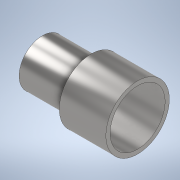
# Autodesk Inventor part: Front Nozzle
Saved by Autodesk Inventor 2021 (Build 250183000, 183)
## iProperties
Created: 2020-04-18
Part Number: Front Nozzle
Material: Generic
Document SubType Name: Modeling
Designer: James
Density: 1 g/cm^3
Appearance: Semi-Polished
Author: James
Autodesk Inventor part; units mm, degrees
ref_plane "YZ Plane" through (0, 0, 0) normal (1, 0, 0) x (0, 1, 0)
ref_plane "XZ Plane" through (0, 0, 0) normal (0, 1, 0) x (-1, 0, 0)
ref_plane "XY Plane" through (0, 0, 0) normal (0, 0, 1) x (1, 0, 0)
sketch "Sketch1" plane through (0, 0, 0) normal (0, 0, 1) x (1, 0, 0)
  line L0 (0, 0) -> (80, 0)
  line L1 (60, 15) -> (60, 11)
  line L2 (60, 11) -> (37, 11)
  line L3 (37, 11) -> (37, 9)
  line L4 (37, 9) -> (62, 9)
  line L5 (62, 9) -> (62, 9)
  line L6 (60, 15) -> (82, 15)
  line L7 (62, 9) -> (62, 13)
  line L8 (62, 13) -> (82, 13)
  line L9 (82, 13) -> (82, 15)
  point P0 (62, 11)
  dimension "d0" = 80
  dimension "d4" = 23
  dimension "d5" = 2
  dimension "d9" = 2
  dimension "d14" = 9
  dimension "d15" = 11
  dimension "d17" = 15
  dimension "d18" = 13
  constraints: 20 end point, 2 horizontal, 2 point on line, 2 vertical
  measures "d0" distance of L0.start L0.end
  measures "d4" distance of L1.end L2.end
  measures "d5" distance of L2.end L3.end
  measures "d9" distance between parallel lines of L5 L1
  measures "d14" distance between parallel lines of L0 L4
  measures "d15" distance between parallel lines of L0 L2
  measures "d17" distance between parallel lines of L0 L6
  measures "d18" distance between parallel lines of L0 L8
revolve "Revolution1" add sketch "Sketch1" angle 360 about axis through (0, 0, 0) along (1, 0, 0)
body "Solid1"
